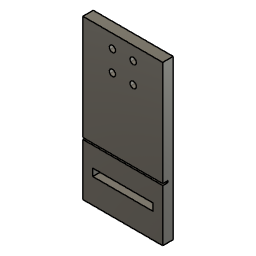
Tube Back Plate v5 (Autodesk Fusion 360 design; units mm, degrees)
Autodesk Fusion 360 part; units mm, degrees
sketch "Sketch1" plane through (0, 0, 0) normal (0, 0, 1) x (1, 0, 0)
  line L0 (0, 0) -> (77, 0)
  line L1 (77, 0) -> (77, 153)
  line L2 (77, 153) -> (0, 153)
  line L3 (0, 153) -> (0, 0)
  circle A0 centre (28.5, 140) radius 3.05
  circle A1 centre (48.5, 140) radius 3.05
  circle A2 centre (28.5, 120) radius 3.05
  circle A3 centre (48.5, 120) radius 3.05
  line L4 (9.5, 31) -> (67.5, 31)
  line L5 (67.5, 31) -> (67.5, 24)
  line L6 (67.5, 24) -> (9.5, 24)
  line L7 (9.5, 24) -> (9.5, 31)
  dimension "d1" = 153
  dimension "d2" = 77
  dimension "d3" = 6.1
  dimension "d4" = 6.1
  dimension "d5" = 6.1
  dimension "d6" = 6.1
  dimension "d7" = 140
  dimension "d8" = 140
  dimension "d9" = 120
  dimension "d10" = 120
  dimension "d11" = 20
  dimension "d12" = 20
  dimension "d13" = 28.5
  dimension "d14" = 28.5
  dimension "d17" = 24
  dimension "d18" = 9.5
  dimension "d19" = 9.5
  dimension "d20" = 7
  constraint horizontal L0
  constraint vertical L1
  constraint horizontal L2
  constraint vertical L3
  constraint coincident L0.start L3.end
  constraint horizontal L4
  constraint vertical L5
  constraint horizontal L6
  constraint vertical L7
  measures "d1" distance of L0.start L2.end
  measures "d2" distance of L1.end L2.end
  measures "d3" diameter of A0
  measures "d4" diameter of A1
  measures "d5" diameter of A2
  measures "d6" diameter of A3
  measures "d7" distance of L0 A0.centre
  measures "d8" distance of L0 A1.centre
  measures "d9" distance of L0 A3.centre
  measures "d10" distance of L0 A2.centre
  measures "d11" distance of A0.centre A1.centre
  measures "d12" distance of A2.centre A3.centre
  measures "d13" distance of L1 A1.centre
  measures "d14" distance of L1 A3.centre
  measures "d17" distance of L0 L6
  measures "d18" distance of L3 L6.end
  measures "d19" distance of L1 L5
  measures "d20" distance of L4.start L6.end
extrude "Extrude1" add sketch "Sketch1" along normal blind 10
sketch "Sketch2" plane through (0, 0, 10) normal (0, 0, 1) x (1, 0, 0)
  circle A0 centre (28.5, 120) radius 3.05
  circle A1 centre (48.5, 120) radius 3.05
  circle A2 centre (48.5, 140) radius 3.05
  circle A3 centre (28.5, 140) radius 3.05
  line L0 (67.5, 24) -> (9.5, 24)
  line L1 (9.5, 24) -> (9.5, 31)
  line L2 (9.5, 31) -> (67.5, 31)
  line L3 (67.5, 31) -> (67.5, 24)
  line L4 (0, 153) -> (0, 0)
  line L5 (0, 0) -> (77, 0)
  line L6 (77, 0) -> (77, 153)
  line L7 (77, 153) -> (0, 153)
  line L8 (0, 51.8) -> (77, 51.8)
  line L9 (77, 51.8) -> (77, 50.2)
  line L10 (77, 50.2) -> (0, 50.2)
  line L11 (0, 50.2) -> (0, 51.8)
  dimension "d21" = 50.2
  dimension "d22" = 51.8
  constraint horizontal L8
  constraint vertical L9
  constraint horizontal L10
  constraint vertical L11
  constraint coincident L6 L9.end
  constraint coincident L4 L8.start
  measures "d21" distance of L5 L10
  measures "d22" distance of L5 L8
extrude "Extrude2" cut sketch "Sketch2" against normal blind 5 contours L4 L6 L8 L9 L10 L11
equation "d4 = d3"
equation "d5 = d3"
equation "d6 = d3"
equation "d8 = d7"
equation "d10 = d9"
equation "d12 = d11"
equation "d14 = d13"
